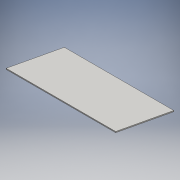
# Autodesk Inventor part: zderzak
Saved by Autodesk Inventor 2016 (Build 200138000, 138)
## iProperties
Created: 2015-11-09
Part Number: zderzak
Material: Ogólny
Document SubType Name: Modeling
Designer: Mrianura
Density: 1 g/cm^3
Appearance: Domyślna
Author: Mrianura
Autodesk Inventor part; units mm, degrees
ref_plane "YZ Plane" through (0, 0, 0) normal (1, 0, 0) x (0, 1, 0)
ref_plane "XZ Plane" through (0, 0, 0) normal (0, 1, 0) x (-1, 0, 0)
ref_plane "XY Plane" through (0, 0, 0) normal (0, 0, 1) x (1, 0, 0)
sketch "Szkic1" plane through (0, 0, 0) normal (1, 0, 0) x (0, 1, 0)
  line L0 (0, 0) -> (0, -1)
  line L1 (0, -1) -> (53.0785, -10.9334)
  line L2 (0, -1) -> (54, -1) construction
  line L3 (53.0785, -10.9334) -> (53.0785, -9.9334)
  line L4 (53.0785, -9.9334) -> (0, 0)
  dimension "d0" = 1
  dimension "d1" = 54
  dimension "d2" = 10.6
  dimension "d3" = 1
  constraints: 10 end point, 2 vertical, 1 equal length, 1 horizontal
  measures "d0" distance of L0.start L0.end
  measures "d1" distance of L0.end L1.end
  measures "d2" angle of L1 L2
  measures "d3" distance of L1.end L3.end
extrude "Wyciągnięcie proste1" add sketch "Szkic1" along normal blind 100
